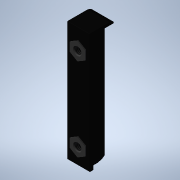
# Autodesk Inventor part: 8116179 MS4-MV-B---(0_high_m)
Saved by Autodesk Inventor 2024.3 (Build 283343000, 343)
## iProperties
Category: PARTsolutions
Company: FESTO
Created: 2025-04-26
Part Number: 8116179 MS4-MV-B---(0_high_m)
Material: Generic
Catalog Web Link: www.cadenas.de
Description: MS4-MV-B_m-module connector
Vendor: FESTO
Document SubType Name: Modeling
Designer: psAdmin
Manufacturer: FESTO
Mass: 1.56044 g
Surface Area: 14.4864 cm^2
Volume: 1.56044 cm^3
Density: 1 g/cm^3
Appearance: PSOLRGB-175-175-175
PSOL_IDENT_0: {$CADENAS_DATA/23d-libs/festo/parts/m/ms4/parts/zubehoer/ms4_mv_b.prj},221 {VTYP=3D},{NB=8116179 MS4
PSOL_IDENT_1: -MV-B---(0_high_m)},{LINA=8116179 MS4-MV-B---(0_high_m)},{NN=MS4-MV-B_m},{DATE=08.04.2024 08:15:04},
PSOL_IDENT_2: {GEOMDATE=08.04.2024 08:15:00},{VERSION=},{LINEID=20},{WBVAR=LODLEVEL,SCREW},{WBNUMERIC=SCREW}  {NB=
PSOL_IDENT_3: 8116179 MS4-MV-B---(0_high_m)},{LINA=8116179 MS4-MV-B---(0_high_m)},{KT=DUMMY},{TNR=8116179},{TYP=MS
PSOL_IDENT_4: 4-MV-B},{VER=2},{LODDEST=mechanical},{LODLEVEL=high},{LODLEVELX='high', 'High', 'medium', 'Medium','
PSOL_IDENT_5: low','Low'},{SCREW=0.0},{SCREW1=0},{X1=0.000}
NB: 8116179 MS4-MV-B---(0_high_m)
NN: MS4-MV-B_m
NT: module connector
NBSYN: $TNR. $TYP.---($SCREW._$LODLEVEL._m)
LINA: 8116179 MS4-MV-B---(0_high_m)
CATALOG: Festo
TNR: 8116179
TYP: MS4-MV-B
VER: 2
LODLEVEL: High
SCREW: 0
X1: 0
SUPPLIER: FESTO
ARTICLENO: 8116179 MS4-MV-B---(0_high_m)
BOMINFO: 8116179 MS4-MV-B---(0_high_m)
CREATOR: CADENAS GmbH
Title: 8116179 MS4-MV-B---(0_high_m)
Author: Cadenas PARTsolutions
Comments: module connector
Autodesk Inventor part; units mm, degrees
sketch "Sketch_1" plane through (0, 0, 0) normal (1, 0, 0) x (0, 1, 0)
  line L0 (22, 5.4) -> (-20.8, 5.4)
  arc A0 (-20.8, 5.4) -> (-21, 5.2) centre (-20.8, 5.2) ccw
  line L1 (-21, 5.2) -> (-21, 1.1788)
  arc A1 (-21, 1.1788) -> (-20.9463, 1.0424) centre (-20.8, 1.1788) ccw
  line L2 (-20.9463, 1.0424) -> (-20.419, 0.477)
  arc A2 (-20.419, 0.477) -> (-19.322, 0) centre (-19.322, 1.5) ccw
  line L3 (-19.322, 0) -> (21.2, 0)
  line L4 (21.2, 0) -> (21.2, -3.3)
  line L5 (21.2, -3.3) -> (21.6171, -3.3)
  line L6 (21.6171, -3.3) -> (22.1063, -2.2509)
  arc A3 (22.1063, -2.2509) -> (22.2, -1.8283) centre (21.2, -1.8283) ccw
  line L7 (22.2, -1.8283) -> (22.2, 5.2)
  arc A4 (22.2, 5.2) -> (22, 5.4) centre (22, 5.2) ccw
  constraints: 16 end point, 10 point on circle, 5 centre point
extrude "Extrusion1" add sketch "Sketch_1" along normal mid plane 8
sketch "Sketch_6" plane through (0, -21.6, 0) normal (0, 1, 0) x (1, 0, 0)
  arc A0 (-1.7301, -0.5774) -> (-2.6364, 0) centre (-2.6364, -1) ccw
  line L0 (-1.7301, -0.5774) -> (-1.2427, -1.6226)
  arc A1 (-1.2427, -1.6226) -> (-0.3364, -2.2) centre (-0.3364, -1.2) ccw
  line L1 (-0.3364, -2.2) -> (0.3364, -2.2)
  arc A2 (0.3364, -2.2) -> (1.2427, -1.6226) centre (0.3364, -1.2) ccw
  line L2 (1.2427, -1.6226) -> (1.7301, -0.5774)
  arc A3 (2.6364, 0) -> (1.7301, -0.5774) centre (2.6364, -1) ccw
  line L3 (2.6364, 0) -> (-2.6364, 0)
  constraints: 8 end point, 8 point on circle, 4 centre point
extrude "Extrusion2" cut sketch "Sketch_6" along normal blind 42.8
sketch "Sketch_9" plane through (0, 0, 0) normal (0, 0, 1) x (1, 0, 0)
  line L0 (-5, -18.3964) -> (-5, -23.2)
  line L1 (-5, -23.2) -> (5, -23.2)
  line L2 (5, -23.2) -> (5, -18.3964)
  line L3 (5, -18.3964) -> (4, -18.3964)
  arc A0 (3.9732, -18.4964) -> (4, -18.3964) centre (3.8, -18.3964) ccw
  line L4 (3.9732, -18.4964) -> (1.8927, -22.1)
  arc A1 (1.7195, -22.2) -> (1.8927, -22.1) centre (1.7195, -22) ccw
  line L5 (1.7195, -22.2) -> (-1.7195, -22.2)
  arc A2 (-1.8927, -22.1) -> (-1.7195, -22.2) centre (-1.7195, -22) ccw
  line L6 (-1.8927, -22.1) -> (-3.9732, -18.4964)
  arc A3 (-4, -18.3964) -> (-3.9732, -18.4964) centre (-3.8, -18.3964) ccw
  line L7 (-4, -18.3964) -> (-5, -18.3964)
  constraints: 16 end point, 8 point on circle, 4 centre point
extrude "Extrusion3" cut sketch "Sketch_9" along normal blind 4
sketch "Sketch_11" plane through (0, 0, 5.4) normal (0, 0, 1) x (1, 0, 0)
  line L0 (-2.75, 13.4123) -> (0, 11.8246)
  line L1 (0, 11.8246) -> (2.75, 13.4123)
  line L2 (2.75, 13.4123) -> (2.75, 16.5877)
  line L3 (2.75, 16.5877) -> (0, 18.1754)
  line L4 (0, 18.1754) -> (-2.75, 16.5877)
  line L5 (-2.75, 16.5877) -> (-2.75, 13.4123)
  constraints: 12 end point
sketch "Sketch_12" plane through (0, 0, 5.4) normal (0, 0, 1) x (1, 0, 0)
  line L0 (-2.75, -16.5877) -> (0, -18.1754)
  line L1 (0, -18.1754) -> (2.75, -16.5877)
  line L2 (2.75, -16.5877) -> (2.75, -13.4123)
  line L3 (2.75, -13.4123) -> (0, -11.8246)
  line L4 (0, -11.8246) -> (-2.75, -13.4123)
  line L5 (-2.75, -13.4123) -> (-2.75, -16.5877)
  constraints: 12 end point
extrude "Extrusion4" add sketch "Sketch_12" along normal blind 0.4
extrude "Extrusion5" add sketch "Sketch_11" along normal blind 0.4
sketch "Sketch_10" plane through (0, 0, 0) normal (1, 0, 0) x (0, 1, 0)
  line L0 (15, 0) -> (15, 5.8)
  line L1 (15, 5.8) -> (16.5, 5.8)
  line L2 (16.5, 5.8) -> (16.2295, 5.5295)
  line L3 (16.2295, 5.5295) -> (16.2295, 4.2705)
  line L4 (16.2295, 4.2705) -> (16.5, 4)
  line L5 (16.5, 4) -> (16.75, 4)
  line L6 (16.75, 4) -> (16.75, 0)
  line L7 (16.75, 0) -> (15, 0)
  line L8 (15, 0) -> (15, 5.8)
  constraints: 18 end point
revolve "Revolution1" cut sketch "Sketch_10" angle 360 about axis through (0, 15, 0) along (0, 0, -1)
thread "Thread1" size "M3x0.5" class "6H" standard "ISO Metric profile" full length
sketch "Sketch_13" plane through (0, 0, 0) normal (1, 0, 0) x (0, 1, 0)
  line L0 (-15, 0) -> (-15, 5.8)
  line L1 (-15, 5.8) -> (-13.5, 5.8)
  line L2 (-13.5, 5.8) -> (-13.7705, 5.5295)
  line L3 (-13.7705, 5.5295) -> (-13.7705, 4.2705)
  line L4 (-13.7705, 4.2705) -> (-13.5, 4)
  line L5 (-13.5, 4) -> (-13.25, 4)
  line L6 (-13.25, 4) -> (-13.25, 0)
  line L7 (-13.25, 0) -> (-15, 0)
  line L8 (-15, 0) -> (-15, 5.8)
  constraints: 18 end point
revolve "Revolution2" cut sketch "Sketch_13" angle 360 about axis through (0, -15, 0) along (0, 0, -1)
thread "Thread2" size "M3x0.5" class "6H" standard "ISO Metric profile" full length
ref_plane "ANBAU_XY" through (0, 0, -15.2) normal (0, -1, 0) x (1, 0, 0)
ref_plane "ANBAU_YZ" through (0, 0, -15.2) normal (1, 0, 0) x (0, 0, 1)
ref_plane "ANBAU_ZX" through (0, 0, -15.2) normal (0, 0, 1) x (0, -1, 0)
ref_plane "ANBAU_2_XY" through (0, 0, -15.2) normal (1, 0, 0) x (0, 0, -1)
ref_plane "ANBAU_2_YZ" through (0, 0, -15.2) normal (0, 0, -1) x (0, 1, 0)
ref_plane "ANBAU_2_ZX" through (0, 0, -15.2) normal (0, 1, 0) x (1, 0, 0)
ref_plane "IP1_XY" through (0, 0, 5.4) normal (0, 0, -1) x (1, 0, 0)
ref_plane "IP1_YZ" through (0, 0, 5.4) normal (1, 0, 0) x (0, -1, 0)
ref_plane "IP1_ZX" through (0, 0, 5.4) normal (0, -1, 0) x (0, 0, -1)
ref_plane "IP_ANBAU_XY" through (0, 0, 0) normal (0, 0, -1) x (1, 0, 0)
ref_plane "IP_ANBAU_YZ" through (0, 0, 0) normal (1, 0, 0) x (0, -1, 0)
ref_plane "IP_ANBAU_ZX" through (0, 0, 0) normal (0, -1, 0) x (0, 0, -1)
ref_plane "IP_ANBAU_2_XY" through (0, 0, -15.2) normal (1, 0, 0) x (0, 0, -1)
ref_plane "IP_ANBAU_2_YZ" through (0, 0, -15.2) normal (0, 0, -1) x (0, 1, 0)
ref_plane "IP_ANBAU_2_ZX" through (0, 0, -15.2) normal (0, 1, 0) x (1, 0, 0)
body "Solid1"
